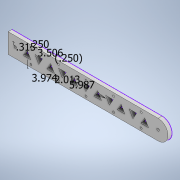
# Autodesk Inventor part: arm_plate_evan
Saved by Autodesk Inventor 2022 (Build 260153000, 153)
## iProperties
Created: 2022-01-24
Part Number: arm_plate_evan
Material: Generic
Document SubType Name: Modeling
Designer: pauly
Density: 1 g/cm^3
Appearance: Default
Author: pauly
Autodesk Inventor part; units mm, degrees
ref_plane "YZ Plane" through (0, 0, 0) normal (1, 0, 0) x (0, 1, 0)
ref_plane "XZ Plane" through (0, 0, 0) normal (0, 1, 0) x (-1, 0, 0)
ref_plane "XY Plane" through (0, 0, 0) normal (0, 0, 1) x (1, 0, 0)
sketch "Sketch1" plane through (0, 0, 0) normal (0, 0, 1) x (1, 0, 0)
  line L0 (0, 0) -> (484.886, 0)
  line L1 (484.886, 63.5) -> (0, 63.5)
  line L2 (0, 63.5) -> (0, 0)
  circle A0 centre (73.914, 53.3905) radius 3.175
  circle A1 centre (162.9664, 53.3905) radius 3.175
  circle A2 centre (252.0188, 53.3868) radius 3.175
  circle A3 centre (341.0712, 53.3868) radius 3.175
  circle A4 centre (430.1236, 53.3868) radius 3.175
  circle A5 centre (73.914, 8.9405) radius 3.175
  circle A6 centre (162.9664, 8.9368) radius 3.175
  circle A7 centre (252.0188, 8.9368) radius 3.175
  circle A8 centre (341.0712, 8.9368) radius 3.175
  circle A9 centre (430.1236, 8.9368) radius 3.175
  line L3 (61.214, 43.0781) -> (73.5873, 21.6469)
  line L4 (48.8407, 21.6469) -> (61.214, 43.0781)
  line L5 (137.414, 43.0781) -> (149.7873, 21.6469)
  line L6 (149.7873, 21.6469) -> (125.0407, 21.6469)
  line L7 (125.0407, 21.6469) -> (137.414, 43.0781)
  line L8 (99.314, 21.6469) -> (86.9407, 43.0781)
  line L9 (86.9407, 43.0781) -> (111.6873, 43.0781)
  line L10 (111.6873, 43.0781) -> (99.314, 21.6469)
  line L11 (48.8407, 21.6469) -> (73.5873, 21.6469)
  line L12 (289.4838, 43.0781) -> (301.8571, 21.6469)
  line L13 (301.8571, 21.6469) -> (277.1105, 21.6469)
  line L14 (277.1105, 21.6469) -> (289.4838, 43.0781)
  line L15 (263.7571, 43.0781) -> (251.3838, 21.6469)
  line L16 (251.3838, 21.6469) -> (239.0105, 43.0781)
  line L17 (239.0105, 43.0781) -> (263.7571, 43.0781)
  line L18 (213.2838, 43.0781) -> (225.6571, 21.6469)
  line L19 (200.9105, 21.6469) -> (225.6571, 21.6469)
  line L20 (200.9105, 21.6469) -> (213.2838, 43.0781)
  line L21 (441.5536, 43.0781) -> (453.9269, 21.6469)
  line L22 (453.9269, 21.6469) -> (429.1803, 21.6469)
  line L23 (429.1803, 21.6469) -> (441.5536, 43.0781)
  line L24 (415.8269, 43.0781) -> (403.4536, 21.6469)
  line L25 (403.4536, 21.6469) -> (391.0803, 43.0781)
  line L26 (391.0803, 43.0781) -> (415.8269, 43.0781)
  line L27 (365.3536, 43.0781) -> (377.7269, 21.6469)
  line L28 (352.9803, 21.6469) -> (377.7269, 21.6469)
  line L29 (352.9803, 21.6469) -> (365.3536, 43.0781)
  line L30 (175.5175, 21.6469) -> (163.1442, 43.0781)
  line L31 (163.1442, 43.0781) -> (187.8909, 43.0781)
  line L32 (187.8909, 43.0781) -> (175.5175, 21.6469)
  line L33 (339.9607, 43.0781) -> (327.5873, 21.6469)
  line L34 (327.5873, 21.6469) -> (315.214, 43.0781)
  line L35 (315.214, 43.0781) -> (339.9607, 43.0781)
  line L36 (15.7817, 31.75) -> (30.4463, 31.75)
  circle A10 centre (23.114, 31.75) radius 4.0005
  circle A11 centre (484.886, 31.75) radius 4.0005
  arc A12 (484.886, 0) -> (484.886, 63.5) centre (484.886, 31.75) ccw
  point P0 (135.1884, 47.8306)
  point P1 (135.1884, 33.5431)
  point P2 (23.114, 19.05)
  point P3 (23.114, 25.4)
  point P4 (287.2582, 33.5431)
  point P5 (439.328, 33.5431)
  dimension "d18" = 44.45
  dimension "d36" = 56.5658
  dimension "d69" = 126.3396
  dimension "d72" = 25.4
  dimension "d12" = 6.35
  dimension "d15" = 89.0524
  dimension "d44" = 6.35
  dimension "d66" = 100.9467
  dimension "d97" = 152.0698
  dimension "d102" = 51.1231
  dimension "d115" = 8.001
  constraints: 74 end point, 13 centre point, 6 horizontal, 2 point on circle, 1 coincident, 1 collinear, 1 midpoint, 1 parallel, 1 tangent, 1 vertical, 40 other
  measures "d12" diameter of A0
  measures "d15" distance of A0.centre A1.centre
  measures "d44" diameter of A1
  measures "d66" distance of L5.end L4.start
  measures "d97" distance of L5.end L12.end
  measures "d102" distance of L19.start L5.end
  measures "d115" diameter of A10
extrude "Extrusion1" add sketch "Sketch1" along normal blind 12.7 contours L2 L1 A12 L0 | L3 L11 L4 | L12 L13 L14 | L15 L16 L17 | L18 L19 L20 | L21 L22 L23 | L24 L25 L26 | L27 L28 L29 | L30 L31 L32 | L33 L34 L35 | A10 L36 | L36 A10 | A11
extrude "Extrusion4" cut sketch "Sketch1" along normal blind 12.7 contours L3 L11 L4
extrude "Extrusion5" cut sketch "Sketch1" along normal blind 12.7 contours L12 L13 L14 | L15 L16 L17 | L18 L19 L20 | L21 L22 L23 | L24 L25 L26 | L27 L28 L29 | L30 L31 L32 | L33 L34 L35
extrude "Extrusion6" cut sketch "Sketch1" along normal blind 25.4 contours A11
extrude "Extrusion7" cut sketch "Sketch1" along normal blind 25.4 contours A10 L36 | L36 A10
body "Solid1"
